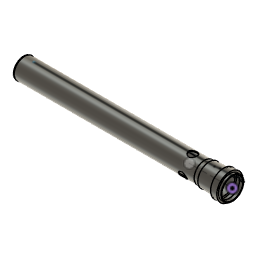
KG ROhr DN50x500 mod v2 (Autodesk Fusion 360 design; units mm, degrees)
Autodesk Fusion 360 part; units mm, degrees
note: some values were not read from the file. Chosen so that the rebuilt part matches the saved one: a direction. Set by a fixed rule: which sketch regions a step uses.
sketch "Skizze1" plane through (0, 0, 0) normal (0, 0, 1) x (1, 0, 0)
  line L0 (-502.8868, 23) -> (-66.7976, 23)
  line L1 (-66.7976, 23) -> (-55.7976, 25.25)
  line L2 (-55.7976, 25.25) -> (-19, 25.25)
  line L3 (-19, 25.25) -> (-19, 29.5)
  line L4 (-19, 29.5) -> (-8, 29.5)
  line L5 (-8, 29.5) -> (-8, 25.5)
  line L6 (-8, 25.5) -> (0, 25.5)
  line L7 (0, 27.5) -> (-6, 27.5)
  line L8 (-6, 27.5) -> (-6, 31.5)
  line L9 (-6, 31.5) -> (-21, 31.5)
  line L10 (-21, 31.5) -> (-21, 27.25)
  line L11 (-21, 27.25) -> (-56, 27.25)
  line L12 (-56, 27.25) -> (-67, 25)
  line L13 (-67, 25) -> (-500.8868, 25)
  line L14 (0, 0) -> (-103.5201, 0)
  line L15 (-502.8868, 23) -> (-502.8868, 24.4641)
  line L16 (-502.8868, 24.4641) -> (-500.8868, 25)
  line L17 (0, 25.5) -> (0, 27.5)
  dimension "d2" = 15
  dimension "d3" = 2
  dimension "d4" = 2
  dimension "d5" = 63
  dimension "d6" = 2
  dimension "d7" = 55
  dimension "d8" = 54.5
  dimension "d10" = 50
  dimension "d12" = 2
  dimension "d13" = 2
  dimension "d14" = 2
  dimension "d15" = 35
  dimension "d16" = 46
  dimension "d17" = 2
  dimension "d18" = 2
  dimension "d19" = 15
  dimension "d21" = 6
  constraint horizontal L0
  constraint parallel L0 L2
  constraint perpendicular L2 L3
  constraint perpendicular L3 L4
  constraint perpendicular L4 L5
  constraint perpendicular L5 L6
  constraint perpendicular L7 L8
  constraint perpendicular L8 L9
  constraint perpendicular L9 L10
  constraint perpendicular L10 L11
  constraint coincident L14.start origin
  constraint parallel L11 L14
  constraint horizontal L13
  constraint parallel L1 L12
  constraint perpendicular L0 L15
  constraint perpendicular L7 L17
  constraint coincident L14.start L17
  measures "d2" distance of L8.end L9.end
  measures "d3" distance of L3 L10
  measures "d4" distance of L5 L8
  measures "d6" distance of L4 L9
  measures "d12" distance of L2 L11
  measures "d13" distance of L1 L12
  measures "d14" distance of L6 L7
  measures "d15" distance of L10.end L11.end
  measures "d16" distance of L10 L12.end
  measures "d17" distance of L0 L13
  measures "d18" distance of L13.end L15
  measures "d19" angle of L13 L16
  measures "d21" distance of L8 L17
revolve "Drehen1" add sketch "Skizze1" angle 360 about axis through (0, 0, 0) along (-1, 0, 0)
sketch "Skizze2" plane through (0, 0, 0) normal (0, 0, 1) x (1, 0, 0)
  line L0 (0, 0) -> (-160, 0) construction
  circle A0 centre (-95, 0) radius 10
  dimension "d23" = 20
  constraint coincident L0.start origin
  constraint horizontal L0
  constraint coincident L0 A0.centre
  measures "d23" diameter of A0
extrude "Extrusion1" cut sketch "Skizze2" along normal up to surface end surface at (-211.6289, 24.9189, 2.0117)
ref_plane "Arbeitsebene1" through (-51.76, 0, 0) normal (0, 0.866025, -0.5) x (-1, 0, 0)
sketch "Skizze3" plane through (0, 0, 0) normal (0, 0.866025, -0.5) x (-1, 0, 0)
  line L0 (0, 0) -> (140, 0)
  spline S0 degree 3 poles (95, 12.9374) (93.7247, 12.9374) (92.3784, 13.1794) (89.9209, 14.081) (88.808, 14.7328) (87.0511, 16.1029) (86.2839, 16.9168) (85.2579, 18.508) (85, 19.2819) (85, 20.5553) (85.2579, 21.1286) (86.2839, 21.9966) (87.0511, 22.2961) (88.808, 22.683) (89.9209, 22.7974) (92.3784, 22.921) (93.7247, 22.9374) (96.2753, 22.9374) (97.6216, 22.921) (100.0791, 22.7974) (101.192, 22.683) (102.9489, 22.2961) (103.7161, 21.9966) (104.7421, 21.1286) (105, 20.5553) (105, 19.2819) (104.7421, 18.508) (103.7161, 16.9168) (102.9489, 16.1029) (101.192, 14.7328) (100.0791, 14.081) (97.6216, 13.1794) (96.2753, 12.9374) (95, 12.9374) knots 0 0 0 0 0.382584 0.382584 0.765167 0.765167 1.147194 1.147194 1.52922 1.52922 1.911247 1.911247 2.293273 2.293273 2.675857 2.675857 3.058441 3.058441 3.441024 3.441024 3.823608 3.823608 4.205634 4.205634 4.587661 4.587661 4.969687 4.969687 5.351714 5.351714 5.734298 5.734298 6.116881 6.116881 6.116881 6.116881
  spline S1 degree 3 poles (95, 14.8431) (96.2719, 14.8431) (97.6172, 15.0731) (100.0759, 15.9379) (101.1907, 16.566) (102.9506, 17.8954) (103.7181, 18.6888) (104.7432, 20.2505) (105, 21.0153) (105, 22.2859) (104.7432, 22.8669) (103.7181, 23.7652) (102.9506, 24.0869) (101.1907, 24.5175) (100.0759, 24.6562) (97.6172, 24.816) (96.2719, 24.8431) (93.7281, 24.8431) (92.3828, 24.816) (89.9241, 24.6562) (88.8093, 24.5175) (87.0494, 24.0869) (86.2819, 23.7652) (85.2568, 22.8669) (85, 22.2859) (85, 21.0153) (85.2568, 20.2505) (86.2819, 18.6888) (87.0494, 17.8954) (88.8093, 16.566) (89.9241, 15.9379) (92.3828, 15.0731) (93.7281, 14.8431) (95, 14.8431) knots 0 0 0 0 0.381558 0.381558 0.763115 0.763115 1.144287 1.144287 1.525459 1.525459 1.90663 1.90663 2.287802 2.287802 2.66936 2.66936 3.050917 3.050917 3.432475 3.432475 3.814033 3.814033 4.195204 4.195204 4.576376 4.576376 4.957548 4.957548 5.338719 5.338719 5.720277 5.720277 6.101835 6.101835 6.101835 6.101835
  spline S2 degree 3 poles (95, 12.9374) (93.7247, 12.9374) (92.3784, 13.1794) (89.9209, 14.081) (88.808, 14.7328) (87.0511, 16.1029) (86.2839, 16.9168) (85.2579, 18.508) (85, 19.2819) (85, 20.5553) (85.2579, 21.1286) (86.2839, 21.9966) (87.0511, 22.2961) (88.808, 22.683) (89.9209, 22.7974) (92.3784, 22.921) (93.7247, 22.9374) (96.2753, 22.9374) (97.6216, 22.921) (100.0791, 22.7974) (101.192, 22.683) (102.9489, 22.2961) (103.7161, 21.9966) (104.7421, 21.1286) (105, 20.5553) (105, 19.2819) (104.7421, 18.508) (103.7161, 16.9168) (102.9489, 16.1029) (101.192, 14.7328) (100.0791, 14.081) (97.6216, 13.1794) (96.2753, 12.9374) (95, 12.9374) knots 0 0 0 0 0.382584 0.382584 0.765167 0.765167 1.147194 1.147194 1.52922 1.52922 1.911247 1.911247 2.293273 2.293273 2.675857 2.675857 3.058441 3.058441 3.441024 3.441024 3.823608 3.823608 4.205634 4.205634 4.587661 4.587661 4.969687 4.969687 5.351714 5.351714 5.734298 5.734298 6.116881 6.116881 6.116881 6.116881
  line L1 (95, 12.9374) -> (95, 0) construction
  circle A0 centre (95, 0) radius 10
  constraint coincident L0.start origin
  constraint horizontal L0
  constraint coincident S0.start S0.end
  constraint coincident L0 L1.end
  constraint perpendicular L0 L1
  constraint coincident L1.end A0.centre
extrude "Extrusion2" cut sketch "Skizze3" along normal up to surface contours L0 A0 | L0 A0 end surface at (-211.6289, 24.9189, 2.0117)
ref_plane "Arbeitsebene2" through (-51.76, 0, 0) normal (0, -0.866025, -0.5) x (-1, 0, 0)
sketch "Skizze4" plane through (0, 0, 0) normal (0, -0.866025, -0.5) x (-1, 0, 0)
  circle A0 centre (97.2112, -0.7111) radius 10
  spline S0 degree 3 poles (95, -22.9374) (93.7247, -22.9374) (92.3784, -22.921) (89.9209, -22.7974) (88.808, -22.683) (87.0511, -22.2961) (86.2839, -21.9966) (85.2579, -21.1286) (85, -20.5553) (85, -19.2819) (85.2579, -18.508) (86.2839, -16.9168) (87.0511, -16.1029) (88.808, -14.7328) (89.9209, -14.081) (92.3784, -13.1794) (93.7247, -12.9374) (96.2753, -12.9374) (97.6216, -13.1794) (100.0791, -14.081) (101.192, -14.7328) (102.9489, -16.1029) (103.7161, -16.9168) (104.7421, -18.508) (105, -19.2819) (105, -20.5553) (104.7421, -21.1286) (103.7161, -21.9966) (102.9489, -22.2961) (101.192, -22.683) (100.0791, -22.7974) (97.6216, -22.921) (96.2753, -22.9374) (95, -22.9374) knots 0 0 0 0 0.382584 0.382584 0.765167 0.765167 1.147194 1.147194 1.52922 1.52922 1.911247 1.911247 2.293273 2.293273 2.675857 2.675857 3.058441 3.058441 3.441024 3.441024 3.823608 3.823608 4.205634 4.205634 4.587661 4.587661 4.969687 4.969687 5.351714 5.351714 5.734298 5.734298 6.116881 6.116881 6.116881 6.116881
  spline S1 degree 3 poles (95, -24.8431) (96.2719, -24.8431) (97.6172, -24.816) (100.0759, -24.6562) (101.1907, -24.5175) (102.9506, -24.0869) (103.7181, -23.7652) (104.7432, -22.8669) (105, -22.2859) (105, -21.0153) (104.7432, -20.2505) (103.7181, -18.6888) (102.9506, -17.8954) (101.1907, -16.566) (100.0759, -15.9379) (97.6172, -15.0731) (96.2719, -14.8431) (93.7281, -14.8431) (92.3828, -15.0731) (89.9241, -15.9379) (88.8093, -16.566) (87.0494, -17.8954) (86.2819, -18.6888) (85.2568, -20.2505) (85, -21.0153) (85, -22.2859) (85.2568, -22.8669) (86.2819, -23.7652) (87.0494, -24.0869) (88.8093, -24.5175) (89.9241, -24.6562) (92.3828, -24.816) (93.7281, -24.8431) (95, -24.8431) knots 0 0 0 0 0.381558 0.381558 0.763115 0.763115 1.144287 1.144287 1.525459 1.525459 1.90663 1.90663 2.287802 2.287802 2.66936 2.66936 3.050917 3.050917 3.432475 3.432475 3.814033 3.814033 4.195204 4.195204 4.576376 4.576376 4.957548 4.957548 5.338719 5.338719 5.720277 5.720277 6.101835 6.101835 6.101835 6.101835
  dimension "d30" = 20
  measures "d30" diameter of A0
extrude "Extrusion3" cut sketch "Skizze4" along normal up to surface contours A0 end surface at (-221.1599, 10.9598, -22.4696)
